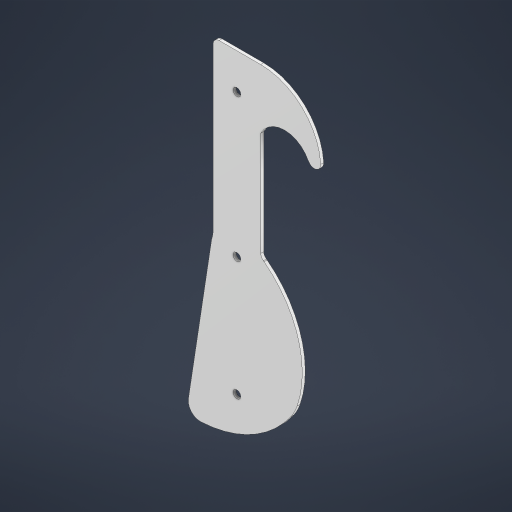
# Autodesk Inventor part: sled
Saved by Autodesk Inventor 2024 (Build 280153000, 153)
## iProperties
Created: 2023-10-27
Part Number: sled
Material: Acetal Resin, White
Document SubType Name: Modeling
Designer: Averey Ku
Density: 1.425 g/cm^3
Appearance: Smooth - White
Author: Averey Ku
Autodesk Inventor part; units mm, degrees
ref_plane "YZ Plane" through (0, 0, 0) normal (1, 0, 0) x (0, 1, 0)
ref_plane "XZ Plane" through (0, 0, 0) normal (0, 1, 0) x (-1, 0, 0)
ref_plane "XY Plane" through (0, 0, 0) normal (0, 0, 1) x (1, 0, 0)
sketch "Sketch1" plane through (0, 0, 0) normal (0, 0, 1) x (1, 0, 0)
  circle A0 centre (-26.9881, -17.2743) radius 2.0955
  circle A1 centre (-26.9881, 46.2257) radius 2.0955
  arc A2 (-46.2652, -39.5915) -> (1.8146, -13.1917) centre (-49.3718, 23.0479) ccw
  arc A3 (5.1303, -6.697) -> (-12.4868, 51.2687) centre (-44.0163, 10.0263) ccw
  line L0 (-52.8546, -32.2756) -> (-40.5161, 47.238)
  arc A4 (1.8146, -13.1917) -> (5.1303, -6.697) centre (-18.9158, 1.4852) ccw
  arc A5 (-52.8546, -32.2756) -> (-46.2652, -39.5915) centre (-46.5797, -33.2493) ccw
  arc A6 (-40.2918, 48.1911) -> (-40.5161, 47.238) centre (-34.2412, 46.2643) ccw
  arc A7 (-12.4868, 51.2687) -> (-12.8478, 51.5252) centre (-16.3434, 46.224) ccw
  circle A8 centre (-26.9881, 122.4257) radius 2.0955
  line L1 (-14.2749, 54.1759) -> (-14.2749, 109.7164)
  line L2 (-39.693, 122.4164) -> (-39.693, 52.0448)
  arc A9 (11.1869, 109.6057) -> (-14.2749, 109.7164) centre (-1.5714, 103.3543) ccw
  arc A10 (11.1869, 109.6057) -> (17.7339, 111.3354) centre (14.2875, 111.125) ccw
  arc A11 (-14.2749, 128.7664) -> (-14.293, 128.7664) centre (-14.293, 89.434) ccw
  arc A12 (-40.2918, 48.1911) -> (-39.693, 52.0448) centre (-52.393, 52.0448) ccw
  arc A13 (-14.2749, 54.1759) -> (-12.8478, 51.5252) centre (-11.0999, 54.1759) ccw
  line L3 (-14.293, 141.4664) -> (-36.518, 141.4664)
  line L4 (-39.693, 138.2914) -> (-39.693, 122.4164)
  arc A14 (17.7339, 111.3354) -> (-14.293, 141.4664) centre (-14.293, 109.3798) ccw
  arc A15 (-36.518, 141.4664) -> (-39.693, 138.2914) centre (-36.518, 138.2914) ccw
  point P0 (-53.9756, -39.4993)
  point P1 (-26.9881, 52.574)
  point P2 (-14.2749, 52.2277)
  point P3 (-39.693, 128.7664)
  point P4 (-39.693, 49.5201)
  dimension "d5" = 4.191
  dimension "d6" = 4.191
  dimension "d7" = 25.4
  dimension "d8" = 6.35
  dimension "d9" = 6.35
  dimension "d11" = 4.191
  dimension "d13" = 25.4
  dimension "d15" = 19.05
  dimension "d18" = 12.7
  dimension "d19" = 3.175
  dimension "d20" = 12.7
  dimension "d21" = 3.175
  constraints: 29 point on circle, 16 centre point, 16 tangent, 10 end point, 5 point on line, 1 equal radius, 1 horizontal, 1 perpendicular, 1 vertical, 4 other
  measures "d5" diameter of A0
  measures "d6" diameter of A1
  measures "d7" radius of A4
  measures "d8" radius of A5
  measures "d9" radius of A6
  measures "d11" diameter of A8
  measures "d13" distance of A11.end point (-39.693, 128.766)
  measures "d15" distance of L1.end A11.end
  measures "d18" radius of A12
  measures "d19" radius of A13
  measures "d20" distance of A11.end L3.start
  measures "d21" radius of A15
extrude "Extrusion1" add sketch "Sketch1" along normal blind 1.5875
body "Solid1"
